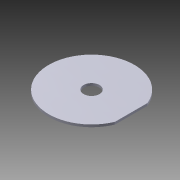
# Autodesk Inventor part: EndCap 108 Cover
Saved by Autodesk Inventor 2015 (Build 190159000, 159)
## iProperties
Created: 2011-09-29
Part Number: EndCap 108 Cover
Document SubType Name: Modeling
Designer: user
Density: 1 g/cm^3
Material: Generic
Appearance: Cool White
Author: user
Autodesk Inventor part; units mm, degrees
ref_plane "YZ Plane" through (0, 0, 0) normal (1, 0, 0) x (0, 1, 0)
ref_plane "XZ Plane" through (0, 0, 0) normal (0, 1, 0) x (-1, 0, 0)
ref_plane "XY Plane" through (0, 0, 0) normal (0, 0, 1) x (1, 0, 0)
sketch "Sketch1" plane through (0, 0, 0) normal (0, 0, 1) x (1, 0, 0)
  circle A0 centre (0, 0) radius 10
  line L0 (50, -20) -> (50, 20)
  arc A1 (49.8462, 20.7692) -> (49.8462, -20.7692) centre (0, 0) ccw
  arc A2 (50, 20) -> (49.8462, 20.7692) centre (48, 20) ccw
  arc A3 (49.8462, -20.7692) -> (50, -20) centre (48, -20) ccw
  point P0 (50, -20.3961)
  point P1 (50, 20.3961)
  dimension "d1" = 20
  dimension "d12" = 50
  dimension "d14" = 54
  constraints: 7 point on circle, 4 centre point, 3 tangent, 2 coincident, 2 end point, 2 point on line, 1 vertical
  measures "d1" diameter of A0
  measures "d12" distance from line of point (0, 0) L0
  measures "d14" radius of A1
extrude "Extrusion3" add sketch "Sketch1" along normal blind 3
body "Solid3"
